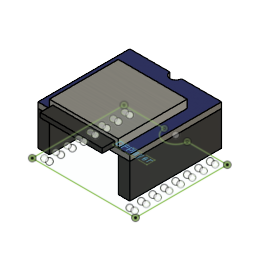
DFPLAYER_MINI_v5 (Autodesk Fusion 360 design; units mm, degrees)
Autodesk Fusion 360 part; units mm, degrees
sketch "Szkic1" plane through (0, 0, 0) normal (0, 0, 1) x (1, 0, 0)
ref_plane "Płaszczyzna konstrukcyjna1" through (0, 8.89, 2.54) normal (0, 0, 1) x (1, 0, 0)
sketch "Szkic2" plane through (0, 0, 2.54) normal (0, 0, 1) x (1, 0, 0)
  line L0 (-10.16, 19.05) -> (-7.62, 19.05)
  line L1 (-7.62, 19.05) -> (-7.62, -1.27)
  line L2 (-7.62, -1.27) -> (-10.16, -1.27)
  line L3 (-10.16, -1.27) -> (-10.16, 19.05)
  line L4 (-2.54, 19.05) -> (-11.43, 19.05)
  line L5 (-8.89, -1.27) -> (-8.89, 2.286) construction
  line L6 (0, 0) -> (0, 6.35) construction
  line L7 (0, 0) -> (0, 6.35) construction
  line L8 (10.16, 19.05) -> (7.62, 19.05)
  line L9 (7.62, -1.27) -> (10.16, -1.27)
  line L10 (8.89, -1.27) -> (8.89, 2.286) construction
  line L11 (7.62, 19.05) -> (7.62, -1.27)
  line L12 (10.16, -1.27) -> (10.16, 19.05)
  point P0 (-8.89, 0)
  point P1 (8.89, 0)
  dimension "d1" = 2.54
  dimension "d2" = 20.32
  constraint horizontal L0
  constraint vertical L1
  constraint horizontal L2
  constraint vertical L3
  constraint collinear L0 L4
  constraint midpoint L2 L5.start
  constraint perpendicular L2 L5
  constraint coincident L5 P0
  constraint coincident L6.start L7.start
  constraint vertical L6
  constraint symmetric L0.start L6 L8.start
  constraint symmetric L0.end L6 L8.end
  constraint symmetric L1.end L6 L9.start
  constraint symmetric L2.end L6 L9.end
  constraint symmetric L5.start L6 L10.start
  constraint symmetric L5.end L6 L10.end
  constraint symmetric P0 L6 P1
  constraint symmetric L7.start L6 origin
  constraint symmetric L7.end L6 L6.end
  measures "d1" distance of L0.start L0.end
  measures "d2" distance of L0.start L2.end
extrude "Wyciągnięcie proste1" add sketch "Szkic2" along normal blind 7.62 makes body 1 at (-7.62, 12.2767, 7.62) makes body 2 at (10.16, 5.5033, 5.08)
sketch "Szkic3" plane through (0, 0, 10.16) normal (0, 0, 1) x (-1, 0, 0)
  line L0 (7.62, -19.05) -> (10.16, -19.05)
  line L1 (10.16, -19.05) -> (10.16, 1.27)
  line L2 (10.16, 1.27) -> (7.62, 1.27)
  line L3 (7.62, 1.27) -> (7.62, -19.05)
  line L4 (-10.16, -19.05) -> (-10.16, 1.27)
  line L5 (-10.16, 1.27) -> (10.16, 1.27)
  line L6 (10.16, 1.27) -> (10.16, -19.05)
  arc A0 (1.27, -19.05) -> (-1.27, -19.05) centre (0, -19.05) ccw
  line L7 (10.16, -19.05) -> (1.27, -19.05)
  line L8 (-1.27, -19.05) -> (-10.16, -19.05)
  dimension "d5" = 2.54
  dimension "d6" = 7.62
  constraint horizontal L7
  constraint vertical L4
  constraint horizontal L5
  constraint vertical L6
  constraint coincident L0.end L1.start
  constraint coincident A0.end L7
  constraint collinear L7 L8
  constraint coincident A0.centre L7
  measures "d5" diameter of A0
  measures "d6" distance of L3 A0.centre
extrude "Wyciągnięcie proste1'" add sketch "Szkic3" along normal blind 1.27 separate body makes body 3 in component "Component"
sketch "Szkic1 (2)" plane through (0, 0, 11.43) normal (0, 0, 1) x (-1, 0, 0) in component "Component'"
  arc A0 (1.27, -19.05) -> (-1.27, -19.05) centre (0, -19.05) ccw
  line L0 (1.27, -19.05) -> (10.16, -19.05)
  line L1 (10.16, -19.05) -> (10.16, 1.27)
  line L2 (10.16, 1.27) -> (-10.16, 1.27)
  line L3 (-10.16, 1.27) -> (-10.16, -19.05)
  line L4 (-10.16, -19.05) -> (-1.27, -19.05)
  line L5 (7.62, 1.27) -> (-7.62, 1.27)
  line L6 (-7.62, 1.27) -> (-7.62, -13.97)
  line L7 (-7.62, -13.97) -> (7.62, -13.97)
  line L8 (7.62, -13.97) -> (7.62, 1.27)
  line L9 (-7.62, -1.2152) -> (-10.16, -1.2152)
  line L10 (7.62, -1.6081) -> (10.16, -1.6081)
  dimension "d9" = 15.24
  dimension "d10" = 15.24
  constraint horizontal L5
  constraint vertical L6
  constraint horizontal L7
  constraint vertical L8
  constraint coincident L2 L5.start
  constraint coincident L6 L9.start
  constraint coincident L3 L9.end
  constraint perpendicular L3 L9
  constraint coincident L8 L10.start
  constraint coincident L1 L10.end
  constraint perpendicular L1 L10
  constraint equal L9 L10
  measures "d9" distance of L5.start L5.end
  measures "d10" distance of L5.start L7.end
extrude "Wyciągnięcie proste1''" add sketch "Szkic1 (2)" along normal blind 1.778 separate body contours L2 L5 L6 L7 L8 makes body 4 in component "Component'"
sketch "Szkic1 (3)" plane through (0, -1.27, 0) normal (0, -1, 0) x (1, 0, 0) in component "Component''"
  line L0 (-7.62, 11.43) -> (7.62, 11.43)
  line L1 (7.62, 11.43) -> (7.62, 13.208)
  line L2 (7.62, 13.208) -> (-7.62, 13.208)
  line L3 (-7.62, 13.208) -> (-7.62, 11.43)
  line L4 (-6.858, 11.43) -> (6.858, 11.43)
  line L5 (6.858, 11.43) -> (6.858, 12.446)
  line L6 (6.858, 12.446) -> (-6.858, 12.446)
  line L7 (-6.858, 12.446) -> (-6.858, 11.43)
  line L8 (-7.62, 12.0457) -> (-6.858, 12.0457)
  line L9 (6.858, 11.938) -> (7.62, 11.938)
  constraint horizontal L4
  constraint vertical L5
  constraint horizontal L6
  constraint vertical L7
  constraint coincident L0 L4.start
  constraint coincident L3 L8.start
  constraint coincident L7 L8.end
  constraint perpendicular L7 L8
  constraint midpoint L5 L9.start
  constraint coincident L1 L9.end
  constraint perpendicular L1 L9
  constraint equal L8 L9
extrude "Wyciągnięcie proste1'''" add sketch "Szkic1 (3)" along normal blind 2.794 separate body contours L0 L4 L5 L6 L7 makes body 5 in component "Component''"
component "Component" placed x (1, 0, 0) y (0, 1, 0) z (0, 0, 1) at (0, 0, 0)
component "Component'" placed x (1, 0, 0) y (0, 1, 0) z (0, 0, 1) at (0, 0, 0) in component "Component"
component "Component''" placed x (1, 0, 0) y (0, 1, 0) z (0, 0, 1) at (0, 0, 0) in component "Component'"
